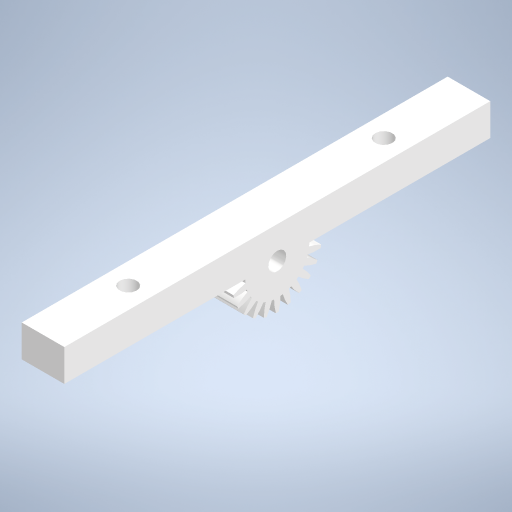
# Autodesk Inventor part: 회전체_3d프린트_1
Saved by Autodesk Inventor 2024 (Build 280153000, 153)
## iProperties
Created: 2024-04-13
Part Number: 회전체_3d프린트_1
Material: ABS 플라스틱
Document SubType Name: Modeling
Designer: kkamin5
Density: 1.06 g/cm^3
Appearance: 매끄러움 - 흰색
Author: kkamin5
Autodesk Inventor part; units mm, degrees
ref_plane "YZ Plane" through (0, 0, 0) normal (1, 0, 0) x (0, 1, 0)
ref_plane "XZ Plane" through (0, 0, 0) normal (0, 1, 0) x (-1, 0, 0)
ref_plane "XY Plane" through (0, 0, 0) normal (0, 0, 1) x (1, 0, 0)
sketch "스케치1" plane through (0, 0, 0) normal (1, 0, 0) x (0, 1, 0)
  circle A0 centre (0, 0) radius 2.1
  circle A1 centre (0, 0) radius 7.5
  line L0 (7.5, 50) -> (-7.5, 50)
  line L1 (-7.5, 50) -> (-7.5, -50)
  line L2 (-7.5, -50) -> (7.5, -50)
  line L3 (7.5, -50) -> (7.5, 50)
  line L4 (7.5, 50) -> (-7.5, -50) construction
  line L5 (-7.5, 50) -> (7.5, -50) construction
  line L6 (0, 50) -> (0, -50)
  point P0 (0, 7.5)
  point P1 (0, -7.5)
  dimension "d0" = 4.2
  dimension "d1" = 15
  dimension "d2" = 100
  constraints: 14 end point, 4 midpoint, 2 centre point, 2 coincident, 2 parallel, 1 horizontal, 1 perpendicular, 1 tangent
  measures "d0" diameter of A0
  measures "d1" diameter of A1
  measures "d2" distance of L1.end L0.end
extrude "돌출1" add sketch "스케치1" along normal mid plane 10 contours A0 L6 A1 | A0 L6 A1 | L6 L0 L3 A1 | A1 L3 L2 L6
sketch "스케치4" plane through (-5, 7.5, 50) normal (0, 1, 0) x (1, 0, 0)
  line L0 (0, 100) -> (10, 100) projected
  point P0 (5, 50)
  point P1 (5, 80)
  point P2 (5, 20)
  point P3 (5, 100)
  dimension "d42" = 60
  dimension "d43" = 20
  constraints: 1 midpoint
  measures "d42" distance of point (5, 20) point (5, 80)
  measures "d43" distance of point (5, 80) point (5, 100)
hole "구멍2" at (0, 7.5, -30) at (0, 7.5, 30) direction (0, -1, 0) diameter 4 end through all
sketch "스케치5" plane through (5, 0, 0) normal (1, 0, 0) x (0, 0, -1)
  circle A0 centre (0, 0) radius 7.5
  line L0 (-0.75, -7.4624) -> (-0.75, -8.8725) construction
  line L1 (-0.75, -8.8725) -> (-0.34, -10.4624) construction
  spline S0 degree 2 poles (-0.75, -7.4624) (-0.75, -8.8725) (-0.34, -10.4624) knots 1 1 1 2 2 2
  line L2 (0, -4.1783) -> (0, -6.6736)
  line L3 (-0.34, -10.4624) -> (0, -10.4624)
  line L4 (-0.75, -7.4624) -> (0, -7.4624)
  line L5 (0, -7.4624) -> (0, -10.4624)
  spline S1 degree 2 poles (0.75, -7.4624) (0.75, -8.8725) (0.34, -10.4624) knots 1 1 1 2 2 2
  line L6 (0.75, -7.4624) -> (0.75, -8.8725) construction
  line L7 (0.75, -8.8725) -> (0.34, -10.4624) construction
  line L8 (0.34, -10.4624) -> (0, -10.4624)
  line L9 (0.75, -7.4624) -> (0, -7.4624)
  circle A1 centre (0, 0) radius 7.5
  circle A2 centre (0, 0) radius 7.5
  line L10 (1.2911, -7.388) -> (1.6716, -8.7458) construction
  line L11 (1.6716, -8.7458) -> (2.4953, -10.1662) construction
  spline S2 degree 2 poles (1.2911, -7.388) (1.6716, -8.7458) (2.4953, -10.1662) knots 1 1 1 2 2 2
  line L12 (1.1273, -4.0234) -> (1.8005, -6.4261)
  line L13 (2.4953, -10.1662) -> (2.8227, -10.0744)
  line L14 (1.2911, -7.388) -> (2.0133, -7.1857)
  line L15 (2.0133, -7.1857) -> (2.8227, -10.0744)
  spline S3 degree 2 poles (2.7355, -6.9833) (3.116, -8.3411) (3.1501, -9.9827) knots 1 1 1 2 2 2
  line L16 (2.7355, -6.9833) -> (3.116, -8.3411) construction
  line L17 (3.116, -8.3411) -> (3.1501, -9.9827) construction
  line L18 (3.1501, -9.9827) -> (2.8227, -10.0744)
  line L19 (2.7355, -6.9833) -> (2.0133, -7.1857)
  circle A3 centre (0, 0) radius 7.5
  line L20 (3.2365, -6.7657) -> (3.9692, -7.9705) construction
  line L21 (3.9692, -7.9705) -> (5.1456, -9.1159) construction
  spline S4 degree 2 poles (3.2365, -6.7657) (3.9692, -7.9705) (5.1456, -9.1159) knots 1 1 1 2 2 2
  line L22 (2.171, -3.57) -> (3.4675, -5.7021)
  line L23 (5.1456, -9.1159) -> (5.4361, -8.9393)
  line L24 (3.2365, -6.7657) -> (3.8773, -6.376)
  line L25 (3.8773, -6.376) -> (5.4361, -8.9393)
  spline S5 degree 2 poles (4.5182, -5.9863) (5.2508, -7.1911) (5.7266, -8.7626) knots 1 1 1 2 2 2
  line L26 (4.5182, -5.9863) -> (5.2508, -7.1911) construction
  line L27 (5.2508, -7.1911) -> (5.7266, -8.7626) construction
  line L28 (5.7266, -8.7626) -> (5.4361, -8.9393)
  line L29 (4.5182, -5.9863) -> (3.8773, -6.376)
  circle A4 centre (0, 0) radius 7.5
  line L30 (4.9419, -5.6416) -> (5.9724, -6.6041) construction
  line L31 (5.9724, -6.6041) -> (7.4142, -7.3896) construction
  spline S6 degree 2 poles (4.9419, -5.6416) (5.9724, -6.6041) (7.4142, -7.3896) knots 1 1 1 2 2 2
  line L32 (3.0537, -2.8519) -> (4.8773, -4.5551)
  line L33 (7.4142, -7.3896) -> (7.6463, -7.1411)
  line L34 (4.9419, -5.6416) -> (5.4538, -5.0935)
  line L35 (5.4538, -5.0935) -> (7.6463, -7.1411)
  spline S7 degree 2 poles (5.9657, -4.5454) (6.9962, -5.5078) (7.8784, -6.8927) knots 1 1 1 2 2 2
  line L36 (5.9657, -4.5454) -> (6.9962, -5.5078) construction
  line L37 (6.9962, -5.5078) -> (7.8784, -6.8927) construction
  line L38 (7.8784, -6.8927) -> (7.6463, -7.1411)
  line L39 (5.9657, -4.5454) -> (5.4538, -5.0935)
  circle A5 centre (0, 0) radius 7.5
  line L40 (6.2807, -4.0991) -> (7.5327, -4.7478) construction
  line L41 (7.5327, -4.7478) -> (9.133, -5.1153) construction
  spline S8 degree 2 poles (6.2807, -4.0991) (7.5327, -4.7478) (9.133, -5.1153) knots 1 1 1 2 2 2
  line L42 (3.7099, -1.9223) -> (5.9254, -3.0703)
  line L43 (9.133, -5.1153) -> (9.2894, -4.8134)
  line L44 (6.2807, -4.0991) -> (6.6258, -3.4332)
  line L45 (6.6258, -3.4332) -> (9.2894, -4.8134)
  spline S9 degree 2 poles (6.9708, -2.7673) (8.2228, -3.416) (9.4458, -4.5115) knots 1 1 1 2 2 2
  line L46 (6.9708, -2.7673) -> (8.2228, -3.416) construction
  line L47 (8.2228, -3.416) -> (9.4458, -4.5115) construction
  line L48 (9.4458, -4.5115) -> (9.2894, -4.8134)
  line L49 (6.9708, -2.7673) -> (6.6258, -3.4332)
  circle A6 centre (0, 0) radius 7.5
  line L50 (7.1537, -2.2526) -> (8.5343, -2.5395) construction
  line L51 (8.5343, -2.5395) -> (10.1744, -2.4615) construction
  spline S10 degree 2 poles (7.1537, -2.2526) (8.5343, -2.5395) (10.1744, -2.4615) knots 1 1 1 2 2 2
  line L52 (4.0909, -0.8501) -> (6.534, -1.3578)
  line L53 (10.1744, -2.4615) -> (10.2436, -2.1286)
  line L54 (7.1537, -2.2526) -> (7.3063, -1.5183)
  line L55 (7.3063, -1.5183) -> (10.2436, -2.1286)
  spline S11 degree 2 poles (7.4589, -0.784) (8.8395, -1.0708) (10.3127, -1.7958) knots 1 1 1 2 2 2
  line L56 (7.4589, -0.784) -> (8.8395, -1.0708) construction
  line L57 (8.8395, -1.0708) -> (10.3127, -1.7958) construction
  line L58 (10.3127, -1.7958) -> (10.2436, -2.1286)
  line L59 (7.4589, -0.784) -> (7.3063, -1.5183)
  circle A7 centre (0, 0) radius 7.5
  line L60 (7.4962, -0.239) -> (8.903, -0.1428) construction
  line L61 (8.903, -0.1428) -> (10.4612, 0.3748) construction
  spline S12 degree 2 poles (7.4962, -0.239) (8.903, -0.1428) (10.4612, 0.3748) knots 1 1 1 2 2 2
  line L62 (4.1686, 0.2851) -> (6.658, 0.4554)
  line L63 (10.4612, 0.3748) -> (10.438, 0.714)
  line L64 (7.4962, -0.239) -> (7.445, 0.5093)
  line L65 (7.445, 0.5093) -> (10.438, 0.714)
  spline S13 degree 2 poles (7.3938, 1.2575) (8.8006, 1.3537) (10.4148, 1.0532) knots 1 1 1 2 2 2
  line L66 (7.3938, 1.2575) -> (8.8006, 1.3537) construction
  line L67 (8.8006, 1.3537) -> (10.4148, 1.0532) construction
  line L68 (10.4148, 1.0532) -> (10.438, 0.714)
  line L69 (7.3938, 1.2575) -> (7.445, 0.5093)
  circle A8 centre (0, 0) radius 7.5
  line L70 (7.2827, 1.7923) -> (8.6113, 2.2645) construction
  line L71 (8.6113, 2.2645) -> (9.9722, 3.1833) construction
  spline S14 degree 2 poles (7.2827, 1.7923) (8.6113, 2.2645) (9.9722, 3.1833) knots 1 1 1 2 2 2
  line L72 (3.9371, 1.3992) -> (6.2883, 2.2349)
  line L73 (9.9722, 3.1833) -> (9.8583, 3.5036)
  line L74 (7.2827, 1.7923) -> (7.0315, 2.499)
  line L75 (7.0315, 2.499) -> (9.8583, 3.5036)
  spline S15 degree 2 poles (6.7804, 3.2057) (8.109, 3.6779) (9.7445, 3.824) knots 1 1 1 2 2 2
  line L76 (6.7804, 3.2057) -> (8.109, 3.6779) construction
  line L77 (8.109, 3.6779) -> (9.7445, 3.824) construction
  line L78 (9.7445, 3.824) -> (9.8583, 3.5036)
  line L79 (6.7804, 3.2057) -> (7.0315, 2.499)
  circle A9 centre (0, 0) radius 7.5
  line L80 (6.5291, 3.6907) -> (7.681, 4.5038) construction
  line L81 (7.681, 4.5038) -> (8.7435, 5.7557) construction
  spline S16 degree 2 poles (6.5291, 3.6907) (7.681, 4.5038) (8.7435, 5.7557) knots 1 1 1 2 2 2
  line L82 (3.4136, 2.4095) -> (5.4521, 3.8485)
  line L83 (8.7435, 5.7557) -> (8.5475, 6.0335)
  line L84 (6.5291, 3.6907) -> (6.0966, 4.3034)
  line L85 (6.0966, 4.3034) -> (8.5475, 6.0335)
  spline S17 degree 2 poles (5.6641, 4.9161) (6.816, 5.7293) (8.3514, 6.3112) knots 1 1 1 2 2 2
  line L86 (5.6641, 4.9161) -> (6.816, 5.7293) construction
  line L87 (6.816, 5.7293) -> (8.3514, 6.3112) construction
  line L88 (8.3514, 6.3112) -> (8.5475, 6.0335)
  line L89 (5.6641, 4.9161) -> (6.0966, 4.3034)
  circle A10 centre (0, 0) radius 7.5
  line L90 (5.2912, 5.3154) -> (6.1811, 6.4092) construction
  line L91 (6.1811, 6.4092) -> (6.8664, 7.9012) construction
  spline S18 degree 2 poles (5.2912, 5.3154) (6.1811, 6.4092) (6.8664, 7.9012) knots 1 1 1 2 2 2
  line L92 (2.6369, 3.2412) -> (4.2116, 5.1768)
  line L93 (6.8664, 7.9012) -> (6.6027, 8.1158)
  line L94 (5.2912, 5.3154) -> (4.7094, 5.7887)
  line L95 (4.7094, 5.7887) -> (6.6027, 8.1158)
  spline S19 degree 2 poles (4.1277, 6.262) (5.0175, 7.3558) (6.339, 8.3304) knots 1 1 1 2 2 2
  line L96 (4.1277, 6.262) -> (5.0175, 7.3558) construction
  line L97 (5.0175, 7.3558) -> (6.339, 8.3304) construction
  line L98 (6.339, 8.3304) -> (6.6027, 8.1158)
  line L99 (4.1277, 6.262) -> (4.7094, 5.7887)
  circle A11 centre (0, 0) radius 7.5
  line L100 (3.6609, 6.5458) -> (4.2227, 7.8391) construction
  line L101 (4.2227, 7.8391) -> (4.4801, 9.4608) construction
  spline S20 degree 2 poles (3.6609, 6.5458) (4.2227, 7.8391) (4.4801, 9.4608) knots 1 1 1 2 2 2
  line L102 (1.6646, 3.8324) -> (2.6588, 6.1211)
  line L103 (4.4801, 9.4608) -> (4.1682, 9.5962)
  line L104 (3.6609, 6.5458) -> (2.973, 6.8446)
  line L105 (2.973, 6.8446) -> (4.1682, 9.5962)
  spline S21 degree 2 poles (2.2851, 7.1434) (2.8469, 8.4367) (3.8564, 9.7317) knots 1 1 1 2 2 2
  line L106 (2.2851, 7.1434) -> (2.8469, 8.4367) construction
  line L107 (2.8469, 8.4367) -> (3.8564, 9.7317) construction
  line L108 (3.8564, 9.7317) -> (4.1682, 9.5962)
  line L109 (2.2851, 7.1434) -> (2.973, 6.8446)
  circle A12 centre (0, 0) radius 7.5
  line L110 (1.7591, 7.2908) -> (1.9511, 8.6877) construction
  line L111 (1.9511, 8.6877) -> (1.7615, 10.3187) construction
  spline S22 degree 2 poles (1.7591, 7.2908) (1.9511, 8.6877) (1.7615, 10.3187) knots 1 1 1 2 2 2
  line L112 (0.5689, 4.1394) -> (0.9087, 6.6114)
  line L113 (1.7615, 10.3187) -> (1.4246, 10.365)
  line L114 (1.7591, 7.2908) -> (1.0161, 7.3929)
  line L115 (1.0161, 7.3929) -> (1.4246, 10.365)
  spline S23 degree 2 poles (0.2731, 7.495) (0.4651, 8.892) (1.0878, 10.4113) knots 1 1 1 2 2 2
  line L116 (0.2731, 7.495) -> (0.4651, 8.892) construction
  line L117 (0.4651, 8.892) -> (1.0878, 10.4113) construction
  line L118 (1.0878, 10.4113) -> (1.4246, 10.365)
  line L119 (0.2731, 7.495) -> (1.0161, 7.3929)
  circle A13 centre (0, 0) radius 7.5
  line L120 (-0.2731, 7.495) -> (-0.4651, 8.892) construction
  line L121 (-0.4651, 8.892) -> (-1.0878, 10.4113) construction
  spline S24 degree 2 poles (-0.2731, 7.495) (-0.4651, 8.892) (-1.0878, 10.4113) knots 1 1 1 2 2 2
  line L122 (-0.5689, 4.1394) -> (-0.9087, 6.6114)
  line L123 (-1.0878, 10.4113) -> (-1.4246, 10.365)
  line L124 (-0.2731, 7.495) -> (-1.0161, 7.3929)
  line L125 (-1.0161, 7.3929) -> (-1.4246, 10.365)
  spline S25 degree 2 poles (-1.7591, 7.2908) (-1.9511, 8.6877) (-1.7615, 10.3187) knots 1 1 1 2 2 2
  line L126 (-1.7591, 7.2908) -> (-1.9511, 8.6877) construction
  line L127 (-1.9511, 8.6877) -> (-1.7615, 10.3187) construction
  line L128 (-1.7615, 10.3187) -> (-1.4246, 10.365)
  line L129 (-1.7591, 7.2908) -> (-1.0161, 7.3929)
  circle A14 centre (0, 0) radius 7.5
  line L130 (-2.2851, 7.1434) -> (-2.8469, 8.4367) construction
  line L131 (-2.8469, 8.4367) -> (-3.8564, 9.7317) construction
  spline S26 degree 2 poles (-2.2851, 7.1434) (-2.8469, 8.4367) (-3.8564, 9.7317) knots 1 1 1 2 2 2
  line L132 (-1.6646, 3.8324) -> (-2.6588, 6.1211)
  line L133 (-3.8564, 9.7317) -> (-4.1682, 9.5962)
  line L134 (-2.2851, 7.1434) -> (-2.973, 6.8446)
  line L135 (-2.973, 6.8446) -> (-4.1682, 9.5962)
  spline S27 degree 2 poles (-3.6609, 6.5458) (-4.2227, 7.8391) (-4.4801, 9.4608) knots 1 1 1 2 2 2
  line L136 (-3.6609, 6.5458) -> (-4.2227, 7.8391) construction
  line L137 (-4.2227, 7.8391) -> (-4.4801, 9.4608) construction
  line L138 (-4.4801, 9.4608) -> (-4.1682, 9.5962)
  line L139 (-3.6609, 6.5458) -> (-2.973, 6.8446)
  circle A15 centre (0, 0) radius 7.5
  line L140 (-4.1277, 6.262) -> (-5.0175, 7.3558) construction
  line L141 (-5.0175, 7.3558) -> (-6.339, 8.3304) construction
  spline S28 degree 2 poles (-4.1277, 6.262) (-5.0175, 7.3558) (-6.339, 8.3304) knots 1 1 1 2 2 2
  line L142 (-2.6369, 3.2412) -> (-4.2116, 5.1768)
  line L143 (-6.339, 8.3304) -> (-6.6027, 8.1158)
  line L144 (-4.1277, 6.262) -> (-4.7094, 5.7887)
  line L145 (-4.7094, 5.7887) -> (-6.6027, 8.1158)
  spline S29 degree 2 poles (-5.2912, 5.3154) (-6.1811, 6.4092) (-6.8664, 7.9012) knots 1 1 1 2 2 2
  line L146 (-5.2912, 5.3154) -> (-6.1811, 6.4092) construction
  line L147 (-6.1811, 6.4092) -> (-6.8664, 7.9012) construction
  line L148 (-6.8664, 7.9012) -> (-6.6027, 8.1158)
  line L149 (-5.2912, 5.3154) -> (-4.7094, 5.7887)
  circle A16 centre (0, 0) radius 7.5
  line L150 (-5.6641, 4.9161) -> (-6.816, 5.7293) construction
  line L151 (-6.816, 5.7293) -> (-8.3514, 6.3112) construction
  spline S30 degree 2 poles (-5.6641, 4.9161) (-6.816, 5.7293) (-8.3514, 6.3112) knots 1 1 1 2 2 2
  line L152 (-3.4136, 2.4095) -> (-5.4521, 3.8485)
  line L153 (-8.3514, 6.3112) -> (-8.5475, 6.0335)
  line L154 (-5.6641, 4.9161) -> (-6.0966, 4.3034)
  line L155 (-6.0966, 4.3034) -> (-8.5475, 6.0335)
  spline S31 degree 2 poles (-6.5291, 3.6907) (-7.681, 4.5038) (-8.7435, 5.7557) knots 1 1 1 2 2 2
  line L156 (-6.5291, 3.6907) -> (-7.681, 4.5038) construction
  line L157 (-7.681, 4.5038) -> (-8.7435, 5.7557) construction
  line L158 (-8.7435, 5.7557) -> (-8.5475, 6.0335)
  line L159 (-6.5291, 3.6907) -> (-6.0966, 4.3034)
  circle A17 centre (0, 0) radius 7.5
  line L160 (-6.7804, 3.2057) -> (-8.109, 3.6779) construction
  line L161 (-8.109, 3.6779) -> (-9.7445, 3.824) construction
  spline S32 degree 2 poles (-6.7804, 3.2057) (-8.109, 3.6779) (-9.7445, 3.824) knots 1 1 1 2 2 2
  line L162 (-3.9371, 1.3992) -> (-6.2883, 2.2349)
  line L163 (-9.7445, 3.824) -> (-9.8583, 3.5036)
  line L164 (-6.7804, 3.2057) -> (-7.0315, 2.499)
  line L165 (-7.0315, 2.499) -> (-9.8583, 3.5036)
  spline S33 degree 2 poles (-7.2827, 1.7923) (-8.6113, 2.2645) (-9.9722, 3.1833) knots 1 1 1 2 2 2
  line L166 (-7.2827, 1.7923) -> (-8.6113, 2.2645) construction
  line L167 (-8.6113, 2.2645) -> (-9.9722, 3.1833) construction
  line L168 (-9.9722, 3.1833) -> (-9.8583, 3.5036)
  line L169 (-7.2827, 1.7923) -> (-7.0315, 2.499)
  circle A18 centre (0, 0) radius 7.5
  line L170 (-7.3938, 1.2575) -> (-8.8006, 1.3537) construction
  line L171 (-8.8006, 1.3537) -> (-10.4148, 1.0532) construction
  spline S34 degree 2 poles (-7.3938, 1.2575) (-8.8006, 1.3537) (-10.4148, 1.0532) knots 1 1 1 2 2 2
  line L172 (-4.1686, 0.2851) -> (-6.658, 0.4554)
  line L173 (-10.4148, 1.0532) -> (-10.438, 0.714)
  line L174 (-7.3938, 1.2575) -> (-7.445, 0.5093)
  line L175 (-7.445, 0.5093) -> (-10.438, 0.714)
  spline S35 degree 2 poles (-7.4962, -0.239) (-8.903, -0.1428) (-10.4612, 0.3748) knots 1 1 1 2 2 2
  line L176 (-7.4962, -0.239) -> (-8.903, -0.1428) construction
  line L177 (-8.903, -0.1428) -> (-10.4612, 0.3748) construction
  line L178 (-10.4612, 0.3748) -> (-10.438, 0.714)
  line L179 (-7.4962, -0.239) -> (-7.445, 0.5093)
  circle A19 centre (0, 0) radius 7.5
  line L180 (-7.4589, -0.784) -> (-8.8395, -1.0708) construction
  line L181 (-8.8395, -1.0708) -> (-10.3127, -1.7958) construction
  spline S36 degree 2 poles (-7.4589, -0.784) (-8.8395, -1.0708) (-10.3127, -1.7958) knots 1 1 1 2 2 2
  line L182 (-4.0909, -0.8501) -> (-6.534, -1.3578)
  line L183 (-10.3127, -1.7958) -> (-10.2436, -2.1286)
  line L184 (-7.4589, -0.784) -> (-7.3063, -1.5183)
  line L185 (-7.3063, -1.5183) -> (-10.2436, -2.1286)
  spline S37 degree 2 poles (-7.1537, -2.2526) (-8.5343, -2.5395) (-10.1744, -2.4615) knots 1 1 1 2 2 2
  line L186 (-7.1537, -2.2526) -> (-8.5343, -2.5395) construction
  line L187 (-8.5343, -2.5395) -> (-10.1744, -2.4615) construction
  line L188 (-10.1744, -2.4615) -> (-10.2436, -2.1286)
  line L189 (-7.1537, -2.2526) -> (-7.3063, -1.5183)
  circle A20 centre (0, 0) radius 7.5
  line L190 (-6.9708, -2.7673) -> (-8.2228, -3.416) construction
  line L191 (-8.2228, -3.416) -> (-9.4458, -4.5115) construction
  spline S38 degree 2 poles (-6.9708, -2.7673) (-8.2228, -3.416) (-9.4458, -4.5115) knots 1 1 1 2 2 2
  line L192 (-3.7099, -1.9223) -> (-5.9254, -3.0703)
  line L193 (-9.4458, -4.5115) -> (-9.2894, -4.8134)
  line L194 (-6.9708, -2.7673) -> (-6.6258, -3.4332)
  line L195 (-6.6258, -3.4332) -> (-9.2894, -4.8134)
  spline S39 degree 2 poles (-6.2807, -4.0991) (-7.5327, -4.7478) (-9.133, -5.1153) knots 1 1 1 2 2 2
  line L196 (-6.2807, -4.0991) -> (-7.5327, -4.7478) construction
  line L197 (-7.5327, -4.7478) -> (-9.133, -5.1153) construction
  line L198 (-9.133, -5.1153) -> (-9.2894, -4.8134)
  line L199 (-6.2807, -4.0991) -> (-6.6258, -3.4332)
  circle A21 centre (0, 0) radius 7.5
  line L200 (-5.9657, -4.5454) -> (-6.9962, -5.5078) construction
  line L201 (-6.9962, -5.5078) -> (-7.8784, -6.8927) construction
  spline S40 degree 2 poles (-5.9657, -4.5454) (-6.9962, -5.5078) (-7.8784, -6.8927) knots 1 1 1 2 2 2
  line L202 (-3.0537, -2.8519) -> (-4.8773, -4.5551)
  line L203 (-7.8784, -6.8927) -> (-7.6463, -7.1411)
  line L204 (-5.9657, -4.5454) -> (-5.4538, -5.0935)
  line L205 (-5.4538, -5.0935) -> (-7.6463, -7.1411)
  spline S41 degree 2 poles (-4.9419, -5.6416) (-5.9724, -6.6041) (-7.4142, -7.3896) knots 1 1 1 2 2 2
  line L206 (-4.9419, -5.6416) -> (-5.9724, -6.6041) construction
  line L207 (-5.9724, -6.6041) -> (-7.4142, -7.3896) construction
  line L208 (-7.4142, -7.3896) -> (-7.6463, -7.1411)
  line L209 (-4.9419, -5.6416) -> (-5.4538, -5.0935)
  circle A22 centre (0, 0) radius 7.5
  line L210 (-4.5182, -5.9863) -> (-5.2508, -7.1911) construction
  line L211 (-5.2508, -7.1911) -> (-5.7266, -8.7626) construction
  spline S42 degree 2 poles (-4.5182, -5.9863) (-5.2508, -7.1911) (-5.7266, -8.7626) knots 1 1 1 2 2 2
  line L212 (-2.171, -3.57) -> (-3.4675, -5.7021)
  line L213 (-5.7266, -8.7626) -> (-5.4361, -8.9393)
  line L214 (-4.5182, -5.9863) -> (-3.8773, -6.376)
  line L215 (-3.8773, -6.376) -> (-5.4361, -8.9393)
  spline S43 degree 2 poles (-3.2365, -6.7657) (-3.9692, -7.9705) (-5.1456, -9.1159) knots 1 1 1 2 2 2
  line L216 (-3.2365, -6.7657) -> (-3.9692, -7.9705) construction
  line L217 (-3.9692, -7.9705) -> (-5.1456, -9.1159) construction
  line L218 (-5.1456, -9.1159) -> (-5.4361, -8.9393)
  line L219 (-3.2365, -6.7657) -> (-3.8773, -6.376)
  circle A23 centre (0, 0) radius 7.5
  line L220 (-2.7355, -6.9833) -> (-3.116, -8.3411) construction
  line L221 (-3.116, -8.3411) -> (-3.1501, -9.9827) construction
  spline S44 degree 2 poles (-2.7355, -6.9833) (-3.116, -8.3411) (-3.1501, -9.9827) knots 1 1 1 2 2 2
  line L222 (-1.1273, -4.0234) -> (-1.8005, -6.4261)
  line L223 (-3.1501, -9.9827) -> (-2.8227, -10.0744)
  line L224 (-2.7355, -6.9833) -> (-2.0133, -7.1857)
  line L225 (-2.0133, -7.1857) -> (-2.8227, -10.0744)
  spline S45 degree 2 poles (-1.2911, -7.388) (-1.6716, -8.7458) (-2.4953, -10.1662) knots 1 1 1 2 2 2
  line L226 (-1.2911, -7.388) -> (-1.6716, -8.7458) construction
  line L227 (-1.6716, -8.7458) -> (-2.4953, -10.1662) construction
  line L228 (-2.4953, -10.1662) -> (-2.8227, -10.0744)
  line L229 (-1.2911, -7.388) -> (-2.0133, -7.1857)
  dimension "d59" = 15
  dimension "d60" = 3
  dimension "d61" = 0.75
  dimension "d62" = 360
  constraints: 276 end point, 46 point on line, 3 symmetric about line, 2 coincident, 2 perpendicular, 2 vertical, 1 centre point, 1 collinear, 1 point on circle, 760 other
  measures "d60" distance between parallel lines of L4 L3
  measures "d61" distance of L4.start L4.end
extrude "돌출3" add sketch "스케치5" against normal blind 10 contours S11 L58 L55 A0 | L55 L53 S10 A0 | S9 L48 L45 A0 | L45 L43 S8 A0 | S7 L38 L35 A0 | L35 L33 S6 A0 | S5 L28 L25 A0 | L25 L23 S4 A0 | S3 L18 L15 A0 | L15 L13 S2 A0 | S1 L8 L5 A0 | L5 L3 S0 A0 | S45 L228 L225 A0 | L225 L223 S44 A0 | S43 L218 L215 A0 | L215 L213 S42 A0 | S41 L208 L205 A0 | L205 L203 S40 A0 | S39 L198 L195 A0 | L195 L193 S38 A0 | S37 L188 L185 A0 | A0 L185 L183 S36
